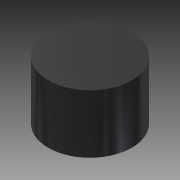
# Autodesk Inventor part: EndEffector
Saved by Autodesk Inventor 2015 (Build 190159000, 159)
## iProperties
Created: 2016-11-08
Part Number: EndEffector
Material: ゴム
Document SubType Name: Modeling
Designer: MobileRoboMaster
Mass: 63.9118 g
Surface Area: 94.2478 cm^2
Volume: 68.7223 cm^3
Density: 0.93 g/cm^3
Appearance: ゴム - 黒 - バージョン 1.1
Author: MobileRoboMaster
Autodesk Inventor part; units mm, degrees
ref_plane "YZ Plane" through (0, 0, 0) normal (1, 0, 0) x (0, 1, 0)
ref_plane "XZ Plane" through (0, 0, 0) normal (0, 1, 0) x (-1, 0, 0)
ref_plane "XY Plane" through (0, 0, 0) normal (0, 0, 1) x (1, 0, 0)
sketch "スケッチ1" plane through (0, 0, 0) normal (0, 0, 1) x (1, 0, 0)
  circle A0 centre (0, 0) radius 25
  dimension "d0" = 50
  constraints: 1 centre point, 1 coincident
  measures "d0" diameter of A0
extrude "押し出し1" add sketch "スケッチ1" along normal mid plane 35
